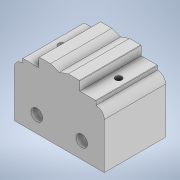
# Autodesk Inventor part: Base soporte tubos
Saved by Autodesk Inventor 2021 (Build 250183000, 183)
## iProperties
Created: 2021-04-30
Part Number: Base soporte tubos
Material: Generic
Document SubType Name: Modeling
Designer: Nelson
Density: 1 g/cm^3
Appearance: Default
Author: Nelson
Autodesk Inventor part; units mm, degrees
ref_plane "YZ Plane" through (0, 0, 0) normal (1, 0, 0) x (0, 1, 0)
ref_plane "XZ Plane" through (0, 0, 0) normal (0, 1, 0) x (-1, 0, 0)
ref_plane "XY Plane" through (0, 0, 0) normal (0, 0, 1) x (1, 0, 0)
sketch "Sketch1" plane through (0, 0, 0) normal (0, 0, 1) x (1, 0, 0)
  line L0 (-110, 0) -> (-110, 112.5)
  arc A0 (-90, 132.5) -> (-110, 112.5) centre (-90, 112.5) ccw
  arc A1 (110, 112.5) -> (90, 132.5) centre (90, 112.5) ccw
  line L1 (110, 112.5) -> (110, 0)
  line L2 (100, 0) -> (110, 0)
  line L3 (-90, 132.5) -> (-90, 142.5)
  line L4 (90, 132.5) -> (90, 142.5)
  line L5 (-50, 142.5) -> (-50, 165)
  line L6 (50, 142.5) -> (50, 165)
  line L7 (-21.6183, 165) -> (0, 157.5)
  line L8 (0, 157.5) -> (21.6183, 165)
  line L9 (-90, 142.5) -> (-50, 142.5)
  line L10 (50, 142.5) -> (90, 142.5)
  line L11 (-110, 0) -> (0, 0)
  line L12 (0, 0) -> (110, 0)
  line L13 (0, 157.5) -> (0, 164) construction
  line L14 (-21.6183, 165) -> (-50, 165)
  line L15 (21.6183, 165) -> (50, 165)
  dimension "d24" = 10
  dimension "d81" = 220
  dimension "d90" = 22.5
  dimension "d91" = 50
  dimension "d92" = 50
  dimension "d101" = 112.5
  dimension "d102" = 20
  dimension "d103" = 20
  dimension "d105" = 15
  dimension "d106" = 30
  dimension "d107" = 30
  constraints: 32 end point, 7 equal length, 5 vertical, 4 horizontal, 4 point on circle, 2 centre point, 2 perpendicular, 1 collinear, 1 equal radius
  measures "d24" distance of L3.start L3.end
  measures "d81" distance between parallel lines of L1 L0
  measures "d90" distance of L5.start L5.end
  measures "d91" distance from line of L11.end L5
  measures "d92" distance from line of L11.end L6
  measures "d101" distance of L0.start L0.end
  measures "d102" radius of A0
  measures "d103" distance between parallel lines of L3 L0
  measures "d105" distance from line of L9 L7.end
  measures "d106" distance from line of L10 L1.start
  measures "d107" distance from line of L9 L0.end
extrude "Extrusion1" add sketch "Sketch1" against normal blind 150
sketch "Sketch4" plane through (-90, 142.5, 0) normal (0, 1, 0) x (1, 0, 0)
  line L0 (0, 0) -> (0, 150) projected
  line L1 (40, 0) -> (0, 0) projected
  line L2 (180, 0) -> (180, 150) projected
  line L3 (180, 0) -> (140, 0) projected
  line L4 (-20, 0) -> (0, 0) projected
  point P0 (90, 0)
  point P1 (20, 75)
  point P2 (160, 75)
  dimension "d62" = 75
  dimension "d63" = 20
  dimension "d64" = 75
  dimension "d65" = 20
  measures "d62" distance from line of L4 point (20, 75)
  measures "d63" distance from line of L0 point (20, 75)
  measures "d64" distance from line of L3 point (160, 75)
  measures "d65" distance from line of L2 point (160, 75)
sketch "Sketch5" plane through (0, 0, 0) normal (0, 0, 1) x (1, 0, 0)
  line L0 (-110, 0) -> (110, 0) projected
  point P0 (0, 0)
  point P1 (-55, 40)
  point P2 (55, 40)
  dimension "d49" = 55
  dimension "d50" = 55
  dimension "d96" = 40
  dimension "d97" = 40
  measures "d49" horizontal distance of point (0, 0) point (-55, 40)
  measures "d50" horizontal distance of point (0, 0) point (55, 40)
  measures "d96" distance from line of L0 point (-55, 40)
  measures "d97" distance from line of L0 point (55, 40)
hole "Hole1" at (-55, 40, 0) at (55, 40, 0) direction (0, 0, -1) diameter 28.4 end through all
hole "Hole2" at (-70, 142.5, -75) at (70, 142.5, -75) direction (0, -1, 0) diameter 15.875 depth 20 tip angle 137
thread "Thread1" size "5/8-11 UNC" class "2B" standard "ANSI Unified Screw Threads" full length
thread "Thread2" size "5/8-11 UNC" class "2B" standard "ANSI Unified Screw Threads" length 70
chamfer "Chamfer1" distance 1 angle 45 4 edges at (-50, 165, -75) (-90, 142.5, -75) (50, 165, -75) (90, 142.5, -75)
equation "\"d92\" = d91"
equation "\"d106\" = d104"
equation "\"d64\" = d62"
equation "\"d65\" = d63"
equation "\"d50\" = d49"
equation "\"d97\" = d96"
equation "\"d36\" = d34"
equation "\"d104\" = 30"
equation "\"d34\" = 75"
body "Solid1"
